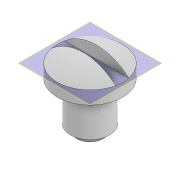
# Autodesk Inventor part: sixth
Saved by Autodesk Inventor 2020 (Build 240168000, 168)
## iProperties
Created: 2021-12-10
Part Number: sixth
Material: Generic
Document SubType Name: Modeling
Designer: NIKHIL VINOD
Density: 1 g/cm^3
Appearance: Default
Author: NIKHIL VINOD
Autodesk Inventor part; units mm, degrees
ref_plane "YZ Plane" through (0, 0, 0) normal (1, 0, 0) x (0, 1, 0)
ref_plane "XZ Plane" through (0, 0, 0) normal (0, 1, 0) x (-1, 0, 0)
ref_plane "XY Plane" through (0, 0, 0) normal (0, 0, 1) x (1, 0, 0)
sketch "Sketch1" plane through (0, 0, 0) normal (0, 0, 1) x (1, 0, 0)
  line L0 (-5, 4.3358) -> (-5, 2.3358)
  line L1 (-5, 2.3358) -> (-3, 2.3358)
  line L2 (-3, 2.3358) -> (-3, -3.6642)
  line L3 (-3, -3.6642) -> (-2, -3.6642)
  line L4 (-2, -3.6642) -> (-2, -4.6642)
  line L5 (-2, -4.6642) -> (0, -4.6642)
  arc A0 (0, 6.3358) -> (-5, 4.3358) centre (0.0877, -1.1334) ccw
  line L6 (0, 6.3358) -> (0, -4.6642)
  point P0 (0, 0)
  dimension "d1" = 2
  dimension "d2" = 2
  dimension "d3" = 6
  dimension "d4" = 1
  dimension "d5" = 1
  constraints: 14 end point, 5 perpendicular, 2 point on circle, 2 vertical, 1 centre point
  measures "d1" distance of L0.start L0.end
  measures "d2" distance of L0.end L1.end
  measures "d3" distance of L1.end L2.end
  measures "d4" distance of L2.end L3.end
  measures "d5" distance of L3.end L4.end
revolve "Revolution1" add sketch "Sketch1" angle 360 about axis through (0, 6.3358, 0) along (0, -1, 0)
ref_plane "Work Plane1" through (0, 4.3358, 0) normal (0, -1, 0) x (1, 0, 0)
sketch "Sketch2" plane through (0, 4.3358, 0) normal (0, -1, 0) x (1, 0, 0)
  line L0 (-5.4528, 1) -> (5.4285, 1)
  line L1 (5.4285, 1) -> (5.4285, -1)
  line L2 (5.4285, -1) -> (-5.4528, -1)
  line L3 (-5.4528, -1) -> (-5.4528, 1)
  point P0 (0, 0)
  dimension "d9" = 2
  dimension "d10" = 1
  constraints: 8 end point, 2 parallel, 1 horizontal, 1 perpendicular
  measures "d9" distance of L2.end L0.start
  measures "d10" distance from line of L0 point (0, 0)
extrude "Extrusion1" cut sketch "Sketch2" against normal blind 10
body "Solid1"
